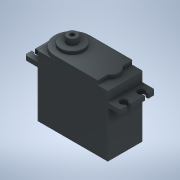
# Autodesk Inventor part: MG996R
Saved by Autodesk Inventor 2020.1 (Build 241239000, 239)
## iProperties
Created: 2021-08-12
Part Number: MG996R
Material: Чугун, литейный
Document SubType Name: Modeling
Designer: User
Density: 7.15 g/cm^3
Appearance: Чугун серый
Author: User
Autodesk Inventor part; units mm, degrees
ref_plane "YZ Plane" through (0, 0, 0) normal (1, 0, 0) x (0, 1, 0)
ref_plane "XZ Plane" through (0, 0, 0) normal (0, 1, 0) x (-1, 0, 0)
ref_plane "XY Plane" through (0, 0, 0) normal (0, 0, 1) x (1, 0, 0)
sketch "Эскиз1" plane through (0, 0, 0) normal (0, 0, 1) x (1, 0, 0)
  line L0 (0, 0) -> (40, 0)
  line L1 (40, 0) -> (40, -36.5)
  line L2 (40, -36.5) -> (0, -36.5)
  line L3 (0, -36.5) -> (0, 0)
  dimension "d0" = 36.5
  dimension "d1" = 40
  constraints: 8 end point, 2 parallel, 1 horizontal, 1 perpendicular
  measures "d0" distance of L2.end L0.start
  measures "d1" distance of L0.start L0.end
extrude "Выдавливание1" add sketch "Эскиз1" along normal blind 19.8
sketch "Эскиз2" plane through (0, 0, 0) normal (0, 1, 0) x (1, 0, 0)
  line L0 (0, 0) -> (0, -19.8) projected
  line L1 (40, 0) -> (0, 0) projected
  circle A0 centre (9.9, -9.9) radius 9.9
  line L2 (9.9, 0) -> (34.3, 0)
  line L3 (34.3, 0) -> (34.3, -19.8)
  line L4 (34.3, -19.8) -> (9.9, -19.8)
  line L5 (9.9, -19.8) -> (9.9, 0)
  line L6 (40, 0) -> (40, -19.8) projected
  circle A1 centre (31.4618, -9.9) radius 5.0382
  point P0 (0, -9.9)
  point P1 (36.5, -9.9)
  point P2 (9.9, 0)
  point P3 (9.9, -19.8)
  point P4 (34.3, -14.0627)
  point P5 (34.3, -5.7373)
  dimension "d4" = 9.9
  dimension "d5" = 9.9
  dimension "d6" = 5.7
  dimension "d7" = 3.5
  constraints: 8 end point, 2 parallel, 1 horizontal, 1 midpoint, 1 perpendicular, 1 point on line, 6 other
  measures "d4" distance of L0.start point (0, -9.9)
  measures "d5" distance of L0.start L2.start
  measures "d6" distance from line of L3 L1.start
  measures "d7" distance from line of L6 point (36.5, -9.9)
extrude "Выдавливание2" add sketch "Эскиз2" along normal blind 2.4 contours A0 L5 | L1 L3 A1 L4 A0 | A0 L5 | A1 L3 | L3 A1
sketch "Эскиз3" plane through (0, 2.4, 0) normal (0, 1, 0) x (1, 0, 0)
  line L0 (0, -9.9) -> (0, -19.8) projected
  circle A0 centre (9.9, -9.9) radius 6.6
  point P0 (0, 0)
  point P1 (9.9, 0)
  dimension "d10" = 13.2
  constraints: 1 centre point
  measures "d10" diameter of A0
extrude "Выдавливание3" add sketch "Эскиз3" along normal blind 1.8
sketch "Эскиз4" plane through (9.9, 4.2, 9.9) normal (0, 1, 0) x (1, 0, 0)
  circle A0 centre (0, 0) radius 2.95
  circle A1 centre (0, 0) radius 1.25
  point P0 (-9.9, 9.9)
  dimension "d13" = 5.9
  dimension "d16" = 2.5
  constraints: 2 centre point, 1 coincident
  measures "d13" diameter of A0
  measures "d16" diameter of A1
extrude "Выдавливание4" add sketch "Эскиз4" along normal blind 3.5
sketch "Эскиз5" plane through (40, -36.5, 0) normal (1, 0, 0) x (0, 0, -1)
  line L0 (-19.8, 0) -> (-19.8, 36.5) projected
  line L1 (0, 0) -> (0, 36.5) projected
  line L2 (-19.8, 28.4) -> (0, 28.4)
  line L3 (0, 28.4) -> (0, 30.8)
  line L4 (0, 30.8) -> (-19.8, 30.8)
  line L5 (-19.8, 30.8) -> (-19.8, 28.4)
  line L6 (0, 0) -> (-19.8, 0) projected
  point P0 (0, 28.4)
  dimension "d17" = 28.4
  dimension "d18" = 2.4
  constraints: 8 end point, 2 parallel, 2 point on line, 1 horizontal, 1 perpendicular
  measures "d17" distance from line of L6 L2.end
  measures "d18" distance from line of L2 L3.end
extrude "Выдавливание5" add sketch "Эскиз5" along normal blind 7 contours L0 L4 L1 L2
sketch "Эскиз6" plane through (0, -36.5, 0) normal (-1, 0, 0) x (0, 0, 1)
  line L0 (19.8, 30.8) -> (0, 30.8) projected
  line L1 (0, 28.4) -> (19.8, 28.4) projected
  line L2 (0, 30.8) -> (19.8, 30.8)
  line L3 (19.8, 30.8) -> (19.8, 28.4)
  line L4 (19.8, 28.4) -> (0, 28.4)
  line L5 (0, 28.4) -> (0, 30.8)
  point P0 (0, 36.5)
  constraints: 8 end point, 2 parallel, 1 horizontal, 1 perpendicular
extrude "Выдавливание6" add sketch "Эскиз6" along normal blind 7
sketch "Эскиз7" plane through (0, -5.7, 19.8) normal (0, 1, 0) x (1, 0, 0)
  line L0 (-7, 0) -> (-7, 19.8) projected
  circle A0 centre (-4, 14.9) radius 2
  circle A1 centre (44, 14.9) radius 2
  line L1 (47, 19.8) -> (47, 0) projected
  circle A2 centre (-4, 4.9) radius 2
  circle A3 centre (44, 4.9) radius 2
  point P0 (0, 19.8)
  point P1 (-7, 9.9)
  dimension "d23" = 4
  dimension "d24" = 5
  dimension "d25" = 3
  dimension "d26" = 4
  dimension "d27" = 48
  dimension "d28" = 3
  dimension "d29" = 4
  dimension "d30" = 5
  constraints: 4 centre point, 1 midpoint
  measures "d23" diameter of A0
  measures "d24" vertical distance of A0.centre point (-7, 9.9)
  measures "d25" distance from line of L0 A0.centre
  measures "d26" diameter of A1
  measures "d27" distance of A1.centre A0.centre
  measures "d28" distance from line of L1 A1.centre
  measures "d29" diameter of A2
  measures "d30" vertical distance of point (-7, 9.9) A2.centre
extrude "Выдавливание7" cut sketch "Эскиз7" against normal blind 10
fillet "Сопряжение1" radius 1 4 edges at (-7, -6.9, 19.8) (-7, -6.9, 0) (47, -6.9, 19.8) (47, -6.9, 0)
chamfer "Фаска1" distance 2 angle 45 4 edges at (20, -36.5, 0) (0, -36.5, 9.9) (20, -36.5, 19.8) (40, -36.5, 9.9)
fillet "Сопряжение3" radius 0.5 10 edges at (0, -21.3, 0) (0, -21.3, 19.8) (0, -2.85, 0) (0, -2.85, 19.8) (40, -21.3, 0) (40, -2.85, 0) (34.3, 1.2, 0) (34.3, 1.2, 19.8) (40, -2.85, 19.8) (40, -21.3, 19.8)
sketch "Эскиз8" plane through (47, -36.5, 0) normal (1, 0, 0) x (0, 0, -1)
  line L0 (-0.5, 30.8) -> (-19.3, 30.8) projected
  line L1 (-19.3, 28.4) -> (-0.5, 28.4) projected
  line L2 (-13.9, 30.8) -> (-15.9, 30.8)
  line L3 (-15.9, 30.8) -> (-15.9, 28.4)
  line L4 (-15.9, 28.4) -> (-13.9, 28.4)
  line L5 (-13.9, 28.4) -> (-13.9, 30.8)
  line L6 (-1, 30.8) -> (-18.8, 30.8) projected
  line L7 (-18.8, 28.4) -> (-1, 28.4) projected
  line L8 (-5.9, 30.8) -> (-3.9, 30.8)
  line L9 (-3.9, 30.8) -> (-3.9, 28.4)
  line L10 (-3.9, 28.4) -> (-5.9, 28.4)
  line L11 (-5.9, 28.4) -> (-5.9, 30.8)
  point P0 (0, 36.5)
  point P1 (-9.9, 30.8)
  point P2 (-14.9, 31.074)
  point P3 (-4.9, 31.074)
  point P4 (-14.9, 30.8)
  dimension "d39" = 5
  dimension "d40" = 1
  dimension "d41" = 4
  dimension "d42" = 4
  dimension "d43" = 6
  constraints: 16 end point, 5 point on line, 4 parallel, 2 horizontal, 2 perpendicular, 1 midpoint
  measures "d39" distance of point (-9.9, 30.8) point (-14.9, 30.8)
  measures "d40" distance of point (-14.9, 30.8) L2.end
  measures "d41" distance of L2.start point (-9.9, 30.8)
  measures "d42" distance of L8.start point (-9.9, 30.8)
  measures "d43" distance of L8.end point (-9.9, 30.8)
extrude "Выдавливание8" cut sketch "Эскиз8" against normal blind 2 contours L9 L1 L11 L0 | L5 L1 L3 L0
sketch "Эскиз9" plane through (-7, -36.5, 0) normal (-1, 0, 0) x (0, 0, 1)
  line L0 (18.8, 30.8) -> (1, 30.8) projected
  line L1 (1, 28.4) -> (18.8, 28.4) projected
  line L2 (5.9, 30.8) -> (3.9, 30.8)
  line L3 (3.9, 30.8) -> (3.9, 28.4)
  line L4 (3.9, 28.4) -> (5.9, 28.4)
  line L5 (5.9, 28.4) -> (5.9, 30.8)
  line L6 (13.9, 30.8) -> (15.9, 30.8)
  line L7 (15.9, 30.8) -> (15.9, 28.4)
  line L8 (15.9, 28.4) -> (13.9, 28.4)
  line L9 (13.9, 28.4) -> (13.9, 30.8)
  point P0 (0, 36.5)
  point P1 (9.9, 30.8)
  dimension "d46" = 4
  dimension "d47" = 6
  dimension "d48" = 4
  dimension "d49" = 6
  constraints: 16 end point, 4 parallel, 4 point on line, 2 horizontal, 2 perpendicular, 1 midpoint
  measures "d46" distance from line of L9 point (9.9, 30.8)
  measures "d47" distance from line of L7 point (9.9, 30.8)
  measures "d48" distance from line of L5 point (9.9, 30.8)
  measures "d49" distance from line of L3 point (9.9, 30.8)
extrude "Выдавливание9" cut sketch "Эскиз9" against normal blind 2 contours L7 L1 L9 L0 | L5 L1 L3 L0
